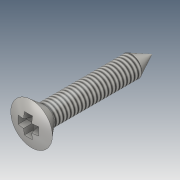
# Autodesk Inventor part: Parafuso do Plug P10
Saved by Autodesk Inventor 2016 (Build 200138000, 138)
## iProperties
Created: 2018-12-01
Part Number: Parafuso do Plug P10
Material: Generic
Document SubType Name: Modeling
Designer: Pedro Mendonça
Density: 1 g/cm^3
Appearance: Aluminum - Dark
Author: Pedro Mendonça
Autodesk Inventor part; units mm, degrees
ref_plane "XZ Plane" through (0, 0, 0) normal (0, 1, 0) x (-1, 0, 0)
sketch "Sketch1" plane through (0, 0, 0) normal (1, 0, 0) x (0, 1, 0)
  circle A0 centre (0, 0) radius 1.25
  dimension "d0" = 2.5
  constraints: 1 centre point, 1 coincident
  measures "d0" diameter of A0
extrude "Extrusion1" add sketch "Sketch1" along normal blind 13
thread "Thread1" size "M2.5x0.45" class "6g" standard "ANSI Metric M Profile" full length
chamfer "Chamfer1" distance 1.25 distance2 2.5 1 edges at (0, -1.25, 0) measured on face at (0, -0.1478, -0.3896)
ref_plane "Work Plane1" through (14.5, 0, 0) normal (1, 0, 0) x (0, 0, -1)
sketch "Sketch2" plane through (14.5, 0, 0) normal (1, 0, 0) x (0, 0, -1)
  circle A0 centre (0, 0) radius 2.5
  dimension "d11" = 5
  constraints: 1 centre point, 1 coincident
  measures "d11" diameter of A0
loft "Loft1" add profiles "Sketch2" section 1 edges at (13, -1.25, 0)
sketch "Sketch3" plane through (0, 0, 0) normal (0, 1, 0) x (-1, 0, 0)
  line L0 (-14.5, -2.5) -> (-14.5, 2.5) construction
  line L1 (-14.5, 0) -> (-15, 0)
  arc A0 (-14.5, 2.5) -> (-15, 0) centre (-8.5, 0) ccw
  line L2 (-14.5, 2.5) -> (-14.5, 0)
  line L3 (3.0248, 0) -> (-18.1485, 0) projected
  point P0 (0, 0)
  dimension "d16" = 0.5
  constraints: 4 end point, 2 point on circle, 1 centre point, 1 collinear, 1 horizontal, 1 midpoint
  measures "d16" distance of L1.end L1.start
revolve "Revolution1" add sketch "Sketch3" angle 360 about axis through (-10, 0, 0) along (1, 0, 0)
ref_plane "Work Plane2" through (15, 0, 0) normal (1, 0, 0) x (0, 1, 0)
sketch "Sketch4" plane through (15, 0, 0) normal (1, 0, 0) x (0, 1, 0)
  line L0 (1.25, 0.5) -> (1.25, -0.5)
  line L1 (-1.25, -0.5) -> (-1.25, 0.5)
  line L2 (0.5, -1.25) -> (-0.5, -1.25)
  line L3 (-0.5, 1.25) -> (0.5, 1.25)
  line L4 (-0.5, -1.25) -> (-0.5, -0.5)
  line L5 (-0.5, 0.5) -> (-0.5, 1.25)
  line L6 (1.25, -0.5) -> (0.5, -0.5)
  line L7 (-0.5, -0.5) -> (-1.25, -0.5)
  line L8 (0.5, 1.25) -> (0.5, 0.5)
  line L9 (0.5, -0.5) -> (0.5, -1.25)
  line L10 (-1.25, 0.5) -> (-0.5, 0.5)
  line L11 (0.5, 0.5) -> (1.25, 0.5)
  dimension "d18" = 2.5
  dimension "d19" = 1
  dimension "d20" = 1
  dimension "d21" = 2.5
  constraints: 24 end point, 10 parallel, 4 perpendicular, 3 horizontal
  measures "d18" distance of L0.end L1.start
  measures "d19" distance of L0.start L0.end
  measures "d20" distance of L3.start L3.end
  measures "d21" distance of L2.end L3.start
extrude "Extrusion2" cut sketch "Sketch4" against normal blind 1 draft -10
body "Solid1"
